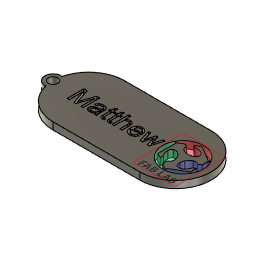
laser name tag v1 (Autodesk Fusion 360 design; units mm, degrees)
Autodesk Fusion 360 part; units mm, degrees
note: some values were not read from the file. Set by a fixed rule: which sketch regions a step uses.
sketch "Sketch1" plane through (0, 0, 0) normal (0, 0, 1) x (1, 0, 0)
  line L0 (15, -15) -> (51.5001, -15)
  arc A0 (51.5001, -15) -> (51.5001, 15) centre (51.5001, 0) ccw
  line L1 (51.5001, 15) -> (15, 15)
  line L2 (0, 0) -> (66.5001, 0) construction
  circle A1 centre (0, 0) radius 2
  line L3 (-3.4999, -0.0257) -> (-3.4999, 9)
  line L4 (15, -13.5) -> (51.5001, -13.5)
  arc A2 (51.5001, -13.5) -> (51.5001, 13.5) centre (51.5001, 0) ccw
  line L5 (51.5001, 13.5) -> (15, 13.5)
  arc A3 (0.4083, 3.4761) -> (0.4083, -3.4761) centre (0, 0) ccw
  arc A4 (15, 15) -> (0.4083, 3.4761) centre (15, 0) ccw
  arc A5 (0.4083, -3.4761) -> (15, -15) centre (15, 0) ccw
  arc A6 (15, 13.5) -> (1.5583, 1.2536) centre (15, 0) ccw
  arc A7 (1.5583, -1.2536) -> (15, -13.5) centre (15, 0) ccw
  dimension "d3" = 30
  dimension "d4" = 7
  dimension "d5" = 70
  constraint tangent L0 A0
  constraint tangent A0 L1
  constraint parallel L0 L1
  constraint tangent L1 A4
  constraint tangent L0 A4
  constraint midpoint A0 L2.end
  constraint horizontal L2
  constraint coincident L3.start A3
  constraint vertical L3
  constraint concentric A4 A5
  constraint coincident L2.start A4
  constraint concentric A0 A2
  constraint tangent L4 A6
  constraint tangent L4 A2
  constraint tangent A2 L5
  constraint tangent L5 A6
  constraint coincident A1 A6.end
  constraint concentric A6 A7
  constraint coincident A1 A7.start
  measures "d3" distance of L0 L1
  measures "d4" diameter of A3
  measures "d5" distance of L2.end L3
extrude "Extrude1" add sketch "Sketch1" along normal blind 3 contours L0 A0 L1 A3 A4 A5 | A1 L4 A2 L5 A6 A7
sketch "Sketch2" plane through (0, 0, 3) normal (0, 0, 1) x (-1, 0, 0)
  circle A0 centre (0, 0) radius 2
  arc A1 (3.4999, 0.0257) -> (-0.4083, 3.4761) centre (0, 0) ccw
  arc A2 (-0.4083, 3.4761) -> (-15, 15) centre (-15, 0) ccw
  line L0 (-15, 15) -> (-51.5001, 15)
  arc A3 (-51.5001, 15) -> (-51.5001, -15) centre (-51.5001, 0) ccw
  line L1 (-51.5001, -15) -> (-15, -15)
  arc A4 (-15, -15) -> (-0.4083, -3.4761) centre (-15, 0) ccw
  arc A5 (-0.4083, -3.4761) -> (3.4999, -0.0257) centre (0, 0) ccw
  line L2 (3.4999, -0.0257) -> (3.4999, 0.0257)
  line L3 (-1.75, 0) -> (-22.5, 0)
  line L4 (-9.4222, 3.5) -> (-9.4222, -3.5)
  line L5 (-9.4222, -3.5) -> (-10.8165, -3.5)
  line L6 (-10.8165, -3.5) -> (-12.4734, 1.4563)
  spline S0 degree 2 poles (-12.4734, 1.4563) (-12.7026, 2.1487) (-12.8076, 2.4925) knots 0 0 0 1 1 1
  spline S1 degree 2 poles (-12.8076, 2.4925) (-12.927, 2.1105) (-13.1801, 1.3704) knots 0 0 0 1 1 1
  line L7 (-13.1801, 1.3704) -> (-14.8561, -3.5)
  line L8 (-14.8561, -3.5) -> (-16.1023, -3.5)
  line L9 (-16.1023, -3.5) -> (-16.1023, 3.5)
  line L10 (-16.1023, 3.5) -> (-15.2094, 3.5)
  line L11 (-15.2094, 3.5) -> (-15.2094, -2.3588)
  line L12 (-15.2094, -2.3588) -> (-13.1753, 3.5)
  line L13 (-13.1753, 3.5) -> (-12.3397, 3.5)
  line L14 (-12.3397, 3.5) -> (-10.3151, -2.4591)
  line L15 (-10.3151, -2.4591) -> (-10.3151, 3.5)
  line L16 (-10.3151, 3.5) -> (-9.4222, 3.5)
  spline S2 degree 2 poles (-20.796, 2.8745) (-20.3186, 3.2804) (-19.8769, 3.4475) knots 0 0 0 1 1 1
  spline S3 degree 2 poles (-19.8769, 3.4475) (-19.4352, 3.6146) (-18.9291, 3.6146) knots 0 0 0 1 1 1
  spline S4 degree 2 poles (-18.9291, 3.6146) (-18.0935, 3.6146) (-17.6446, 3.2063) knots 0 0 0 1 1 1
  spline S5 degree 2 poles (-17.6446, 3.2063) (-17.1958, 2.7981) (-17.1958, 2.163) knots 0 0 0 1 1 1
  spline S6 degree 2 poles (-17.1958, 2.163) (-17.1958, 1.7906) (-17.3653, 1.4826) knots 0 0 0 1 1 1
  spline S7 degree 2 poles (-17.3653, 1.4826) (-17.5348, 1.1746) (-17.8093, 0.9884) knots 0 0 0 1 1 1
  spline S8 degree 2 poles (-17.8093, 0.9884) (-18.0839, 0.8022) (-18.4277, 0.7067) knots 0 0 0 1 1 1
  spline S9 degree 2 poles (-18.4277, 0.7067) (-18.6808, 0.6398) (-19.1917, 0.5778) knots 0 0 0 1 1 1
  spline S10 degree 2 poles (-19.1917, 0.5778) (-20.2326, 0.4536) (-20.7244, 0.2817) knots 0 0 0 1 1 1
  spline S11 degree 2 poles (-20.7244, 0.2817) (-20.7292, 0.105) (-20.7292, 0.0573) knots 0 0 0 1 1 1
  spline S12 degree 2 poles (-20.7292, 0.0573) (-20.7292, -0.4679) (-20.4857, -0.6828) knots 0 0 0 1 1 1
  spline S13 degree 2 poles (-20.4857, -0.6828) (-20.1562, -0.9741) (-19.5068, -0.9741) knots 0 0 0 1 1 1
  spline S14 degree 2 poles (-19.5068, -0.9741) (-18.9004, -0.9741) (-18.6115, -0.7616) knots 0 0 0 1 1 1
  spline S15 degree 2 poles (-18.6115, -0.7616) (-18.3226, -0.5491) (-18.1842, -0.0095) knots 0 0 0 1 1 1
  line L17 (-18.1842, -0.0095) -> (-17.3438, -0.1241)
  spline S16 degree 2 poles (-17.3438, -0.1241) (-17.4584, -0.6637) (-17.721, -0.9956) knots 0 0 0 1 1 1
  spline S17 degree 2 poles (-17.721, -0.9956) (-17.9836, -1.3274) (-18.4802, -1.5065) knots 0 0 0 1 1 1
  spline S18 degree 2 poles (-18.4802, -1.5065) (-18.9768, -1.6855) (-19.631, -1.6855) knots 0 0 0 1 1 1
  spline S19 degree 2 poles (-19.631, -1.6855) (-20.2804, -1.6855) (-20.6862, -1.5327) knots 0 0 0 1 1 1
  spline S20 degree 2 poles (-20.6862, -1.5327) (-21.0921, -1.3799) (-21.2831, -1.1484) knots 0 0 0 1 1 1
  spline S21 degree 2 poles (-21.2831, -1.1484) (-21.4741, -0.9168) (-21.5505, -0.5634) knots 0 0 0 1 1 1
  spline S22 degree 2 poles (-21.5505, -0.5634) (-21.5935, -0.3438) (-21.5935, 0.2292) knots 0 0 0 1 1 1
  line L18 (-21.5935, 0.2292) -> (-21.5935, 1.1)
  spline S23 degree 2 poles (-21.6484, 2.8912) (-21.7033, 3.2087) (-21.8656, 3.5) knots 0 0 0 1 1 1
  line L19 (-21.8656, 3.5) -> (-20.9679, 3.5)
  spline S24 degree 2 poles (-20.9679, 3.5) (-20.8342, 3.2326) (-20.796, 2.8745) knots 0 0 0 1 1 1
  spline S25 degree 2 poles (-20.7244, 0.955) (-20.2565, 1.146) (-19.3206, 1.2797) knots 0 0 0 1 1 1
  spline S26 degree 2 poles (-19.3206, 1.2797) (-18.7906, 1.3561) (-18.5709, 1.4516) knots 0 0 0 1 1 1
  spline S27 degree 2 poles (-18.5709, 1.4516) (-18.3513, 1.5471) (-18.2319, 1.7309) knots 0 0 0 1 1 1
  spline S28 degree 2 poles (-18.2319, 1.7309) (-18.1126, 1.9147) (-18.1126, 2.1392) knots 0 0 0 1 1 1
  spline S29 degree 2 poles (-18.1126, 2.1392) (-18.1126, 2.4829) (-18.3728, 2.7121) knots 0 0 0 1 1 1
  spline S30 degree 2 poles (-18.3728, 2.7121) (-18.633, 2.9413) (-19.1344, 2.9413) knots 0 0 0 1 1 1
  spline S31 degree 2 poles (-19.1344, 2.9413) (-19.631, 2.9413) (-20.0177, 2.7241) knots 0 0 0 1 1 1
  spline S32 degree 2 poles (-20.0177, 2.7241) (-20.4045, 2.5068) (-20.5859, 2.1296) knots 0 0 0 1 1 1
  line L20 (-20.7244, 1.1) -> (-20.7244, 0.955)
  line L21 (-24.8022, 2.7312) -> (-24.9263, 3.4905)
  spline S33 degree 2 poles (-24.9263, 3.4905) (-24.5634, 3.5668) (-24.2769, 3.5668) knots 0 0 0 1 1 1
  spline S34 degree 2 poles (-24.2769, 3.5668) (-23.809, 3.5668) (-23.5512, 3.4188) knots 0 0 0 1 1 1
  spline S35 degree 2 poles (-23.5512, 3.4188) (-23.2933, 3.2708) (-23.1883, 3.0297) knots 0 0 0 1 1 1
  spline S36 degree 2 poles (-23.1883, 3.0297) (-23.0832, 2.7885) (-23.0832, 2.015) knots 0 0 0 1 1 1
  line L22 (-23.0832, 2.015) -> (-23.0832, -0.9025)
  line L23 (-23.0832, -0.9025) -> (-22.4529, -0.9025)
  line L24 (-22.4529, -0.9025) -> (-22.4529, -1.5709)
  line L25 (-22.4529, -1.5709) -> (-23.0832, -1.5709)
  line L26 (-23.0832, -1.5709) -> (-23.0832, -2.8267)
  line L27 (-23.0832, -2.8267) -> (-23.9379, -3.3424)
  line L28 (-23.9379, -3.3424) -> (-23.9379, -1.5709)
  line L29 (-23.9379, -1.5709) -> (-24.8022, -1.5709)
  line L30 (-24.8022, -1.5709) -> (-24.8022, -0.9025)
  line L31 (-24.8022, -0.9025) -> (-23.9379, -0.9025)
  line L32 (-23.9379, -0.9025) -> (-23.9379, 2.0628)
  spline S37 degree 2 poles (-23.9379, 2.0628) (-23.9379, 2.4304) (-23.9833, 2.5355) knots 0 0 0 1 1 1
  spline S38 degree 2 poles (-23.9833, 2.5355) (-24.0286, 2.6405) (-24.1313, 2.7026) knots 0 0 0 1 1 1
  spline S39 degree 2 poles (-24.1313, 2.7026) (-24.234, 2.7647) (-24.425, 2.7647) knots 0 0 0 1 1 1
  spline S40 degree 2 poles (-24.425, 2.7647) (-24.5682, 2.7647) (-24.8022, 2.7312) knots 0 0 0 1 1 1
  line L33 (-27.5191, 2.7312) -> (-27.6432, 3.4905)
  spline S41 degree 2 poles (-27.6432, 3.4905) (-27.2804, 3.5668) (-26.9939, 3.5668) knots 0 0 0 1 1 1
  spline S42 degree 2 poles (-26.9939, 3.5668) (-26.5259, 3.5668) (-26.2681, 3.4188) knots 0 0 0 1 1 1
  spline S43 degree 2 poles (-26.2681, 3.4188) (-26.0102, 3.2708) (-25.9052, 3.0297) knots 0 0 0 1 1 1
  spline S44 degree 2 poles (-25.9052, 3.0297) (-25.8001, 2.7885) (-25.8001, 2.015) knots 0 0 0 1 1 1
  line L34 (-25.8001, 2.015) -> (-25.8001, -0.9025)
  line L35 (-25.8001, -0.9025) -> (-25.1698, -0.9025)
  line L36 (-25.1698, -0.9025) -> (-25.1698, -1.5709)
  line L37 (-25.1698, -1.5709) -> (-25.8001, -1.5709)
  line L38 (-25.8001, -1.5709) -> (-25.8001, -2.8267)
  line L39 (-25.8001, -2.8267) -> (-26.6548, -3.3424)
  line L40 (-26.6548, -3.3424) -> (-26.6548, -1.5709)
  line L41 (-26.6548, -1.5709) -> (-27.5191, -1.5709)
  line L42 (-27.5191, -1.5709) -> (-27.5191, -0.9025)
  line L43 (-27.5191, -0.9025) -> (-26.6548, -0.9025)
  line L44 (-26.6548, -0.9025) -> (-26.6548, 2.0628)
  spline S45 degree 2 poles (-26.6548, 2.0628) (-26.6548, 2.4304) (-26.7002, 2.5355) knots 0 0 0 1 1 1
  spline S46 degree 2 poles (-26.7002, 2.5355) (-26.7456, 2.6405) (-26.8482, 2.7026) knots 0 0 0 1 1 1
  spline S47 degree 2 poles (-26.8482, 2.7026) (-26.9509, 2.7647) (-27.1419, 2.7647) knots 0 0 0 1 1 1
  spline S48 degree 2 poles (-27.1419, 2.7647) (-27.2851, 2.7647) (-27.5191, 2.7312) knots 0 0 0 1 1 1
  line L45 (-28.3595, 3.5) -> (-28.3595, -3.5)
  line L46 (-28.3595, -3.5) -> (-29.219, -3.5)
  line L47 (-29.219, -3.5) -> (-29.219, -0.9884)
  spline S49 degree 2 poles (-29.219, -0.9884) (-29.8206, -1.6855) (-30.7374, -1.6855) knots 0 0 0 1 1 1
  spline S50 degree 2 poles (-30.7374, -1.6855) (-31.3008, -1.6855) (-31.7162, -1.4635) knots 0 0 0 1 1 1
  spline S51 degree 2 poles (-31.7162, -1.4635) (-32.1317, -1.2415) (-32.3107, -0.8499) knots 0 0 0 1 1 1
  spline S52 degree 2 poles (-32.3107, -0.8499) (-32.4898, -0.4584) (-32.4898, 0.2865) knots 0 0 0 1 1 1
  line L48 (-32.4898, 0.2865) -> (-32.4898, 3.5)
  line L49 (-32.4898, 3.5) -> (-31.6303, 3.5)
  line L50 (-31.6303, 3.5) -> (-31.6303, 0.2865)
  spline S53 degree 2 poles (-31.6303, 0.2865) (-31.6303, -0.3581) (-31.351, -0.6518) knots 0 0 0 1 1 1
  spline S54 degree 2 poles (-31.351, -0.6518) (-31.0716, -0.9454) (-30.5607, -0.9454) knots 0 0 0 1 1 1
  spline S55 degree 2 poles (-30.5607, -0.9454) (-30.1787, -0.9454) (-29.8421, -0.7473) knots 0 0 0 1 1 1
  spline S56 degree 2 poles (-29.8421, -0.7473) (-29.5055, -0.5491) (-29.3622, -0.2101) knots 0 0 0 1 1 1
  spline S57 degree 2 poles (-29.3622, -0.2101) (-29.219, 0.1289) (-29.219, 0.7258) knots 0 0 0 1 1 1
  line L51 (-29.219, 0.7258) -> (-29.219, 3.5)
  line L52 (-29.219, 3.5) -> (-28.3595, 3.5)
  line L53 (-37.2694, 1.867) -> (-38.1576, 1.9768)
  spline S58 degree 2 poles (-38.1576, 1.9768) (-37.9475, 2.7551) (-37.3793, 3.1849) knots 0 0 0 1 1 1
  spline S59 degree 2 poles (-37.3793, 3.1849) (-36.8111, 3.6146) (-35.9277, 3.6146) knots 0 0 0 1 1 1
  spline S60 degree 2 poles (-35.9277, 3.6146) (-34.8151, 3.6146) (-34.1634, 2.9294) knots 0 0 0 1 1 1
  spline S61 degree 2 poles (-34.1634, 2.9294) (-33.5116, 2.2442) (-33.5116, 1.0075) knots 0 0 0 1 1 1
  spline S62 degree 2 poles (-33.5116, 1.0075) (-33.5116, -0.2722) (-34.1705, -0.9789) knots 0 0 0 1 1 1
  spline S63 degree 2 poles (-34.1705, -0.9789) (-34.8295, -1.6855) (-35.8799, -1.6855) knots 0 0 0 1 1 1
  spline S64 degree 2 poles (-35.8799, -1.6855) (-36.897, -1.6855) (-37.5416, -0.9932) knots 0 0 0 1 1 1
  spline S65 degree 2 poles (-37.5416, -0.9932) (-38.1862, -0.3008) (-38.1862, 0.955) knots 0 0 0 1 1 1
  spline S66 degree 2 poles (-38.1862, 0.955) (-38.1862, 1.0314) (-38.1814, 1.1842) knots 0 0 0 1 1 1
  spline S67 degree 2 poles (-34.3997, 1.1842) (-34.4475, 2.0198) (-34.8724, 2.4638) knots 0 0 0 1 1 1
  spline S68 degree 2 poles (-34.8724, 2.4638) (-35.2974, 2.9079) (-35.9325, 2.9079) knots 0 0 0 1 1 1
  spline S69 degree 2 poles (-35.9325, 2.9079) (-36.4052, 2.9079) (-36.7394, 2.6596) knots 0 0 0 1 1 1
  spline S70 degree 2 poles (-36.7394, 2.6596) (-37.0737, 2.4113) (-37.2694, 1.867) knots 0 0 0 1 1 1
  spline S71 degree 2 poles (-37.279, 0.4775) (-37.2217, -0.1623) (-36.9543, -0.4823) knots 0 0 0 1 1 1
  spline S72 degree 2 poles (-36.9543, -0.4823) (-36.5437, -0.9789) (-35.8895, -0.9789) knots 0 0 0 1 1 1
  spline S73 degree 2 poles (-35.8895, -0.9789) (-35.2974, -0.9789) (-34.8939, -0.5825) knots 0 0 0 1 1 1
  spline S74 degree 2 poles (-34.8939, -0.5825) (-34.4905, -0.1862) (-34.4475, 0.4775) knots 0 0 0 1 1 1
  line L54 (-40.1726, 3.5) -> (-38.6207, -1.5709)
  line L55 (-38.6207, -1.5709) -> (-39.5089, -1.5709)
  line L56 (-39.5089, -1.5709) -> (-40.3158, 1.3561)
  line L57 (-40.3158, 1.3561) -> (-40.6166, 2.4447)
  spline S75 degree 2 poles (-40.6166, 2.4447) (-40.6357, 2.3636) (-40.8793, 1.399) knots 0 0 0 1 1 1
  line L58 (-40.8793, 1.399) -> (-41.6862, -1.5709)
  line L59 (-41.6862, -1.5709) -> (-42.5696, -1.5709)
  line L60 (-42.5696, -1.5709) -> (-43.3288, 1.3704)
  line L61 (-43.3288, 1.3704) -> (-43.5819, 2.3397)
  line L62 (-43.5819, 2.3397) -> (-43.8731, 1.3608)
  line L63 (-43.8731, 1.3608) -> (-44.7422, -1.5709)
  line L64 (-44.7422, -1.5709) -> (-45.5778, -1.5709)
  line L65 (-45.5778, -1.5709) -> (-43.9925, 3.5)
  line L66 (-43.9925, 3.5) -> (-43.0996, 3.5)
  line L67 (-43.0996, 3.5) -> (-42.2926, 0.4632)
  line L68 (-42.2926, 0.4632) -> (-42.0969, -0.4011)
  line L69 (-42.0969, -0.4011) -> (-41.0703, 3.5)
  line L70 (-41.0703, 3.5) -> (-40.1726, 3.5)
  line L71 (-20.7244, 1.1) -> (-21.5935, 1.1)
  line L72 (-21.5935, 1.4) -> (-20.7225, 1.4)
  spline S76 degree 2 poles (-20.5859, 2.1296) (-20.7081, 1.8726) (-20.7225, 1.4) knots 0 0 0 0.88234 0.88234 0.88234
  spline S77 degree 2 poles (-21.5935, 1.4) (-21.594, 2.577) (-21.6484, 2.8912) knots 0.010398 0.010398 0.010398 1 1 1
  line L73 (-35.9, 0.4775) -> (-35.9, 1.1842)
  line L74 (-35.7, 1.1842) -> (-35.7, 0.4775)
  line L75 (-34.4475, 0.4775) -> (-35.7, 0.4775)
  line L76 (-35.9, 0.4775) -> (-37.279, 0.4775)
  line L77 (-38.1814, 1.1842) -> (-35.9, 1.1842)
  line L78 (-35.7, 1.1842) -> (-34.3997, 1.1842)
  constraint horizontal L71
  constraint horizontal L72
  constraint vertical L73
  constraint vertical L74
  constraint collinear L75 L76
  constraint coincident L74.start L77
  constraint collinear L77 L78
extrude "Extrude2" cut sketch "Sketch2" against normal blind 3 contours L3 L4 L5 L6 L14 L15 | L3 L4 L15 L16 | L3 L6 S0 S1 L7 L12 L13 L14 | L3 L7 L8 L9 L11 L12 | L3 L9 L10 L11 | L3 S12 S13 S14 S15 L17 S16 S17 S18 S19 S20 S21 S22 | L3 S2 S3 S4 S5 S6 S7 S8 S9 S10 S11 S12 S22 L18 S23 L19 S24 S25 S26 S27 S28 S29 S30 S31 S32 L20 L71 L72 S76 S77 | L21 S33 S34 S35 S36 L22 L23 L24 L25 L26 L27 L28 L29 L30 L31 L32 S37 S38 S39 S40 | L33 S41 S42 S43 S44 L34 L35 L36 L37 L38 L39 L40 L41 L42 L43 L44 S45 S46 S47 S48 | L45 L46 L47 S49 S50 S51 S52 L48 L49 L50 S53 S54 S55 S56 S57 L51 L52 | L53 S58 S59 S60 S61 S62 S63 S64 S65 S66 S67 S68 S69 S70 S71 S72 S73 S74 L73 L74 L75 L76 L77 L78 | L54 L55 L56 L57 S75 L58 L59 L60 L61 L62 L63 L64 L65 L66 L67 L68 L69 L70
sketch "Sketch3" plane through (0, 0, 3) normal (0, 0, 1) x (-1, 0, 0)
  spline S0 degree 2 poles (-29.3622, -0.2101) (-29.219, 0.1289) (-29.219, 0.7258) knots 0 0 0 1 1 1
  line L0 (-29.219, 0.7258) -> (-29.219, 3.5)
  line L1 (-29.219, 3.5) -> (-28.3595, 3.5)
  line L2 (-28.3595, 3.5) -> (-28.3595, -3.5)
  line L3 (-28.3595, -3.5) -> (-29.219, -3.5)
  line L4 (-29.219, -3.5) -> (-29.219, -0.9884)
  spline S1 degree 2 poles (-29.219, -0.9884) (-29.8206, -1.6855) (-30.7374, -1.6855) knots 0 0 0 1 1 1
  spline S2 degree 2 poles (-30.7374, -1.6855) (-31.3008, -1.6855) (-31.7162, -1.4635) knots 0 0 0 1 1 1
  spline S3 degree 2 poles (-31.7162, -1.4635) (-32.1317, -1.2415) (-32.3107, -0.8499) knots 0 0 0 1 1 1
  spline S4 degree 2 poles (-32.3107, -0.8499) (-32.4898, -0.4584) (-32.4898, 0.2865) knots 0 0 0 1 1 1
  line L5 (-32.4898, 0.2865) -> (-32.4898, 3.5)
  line L6 (-32.4898, 3.5) -> (-31.6303, 3.5)
  line L7 (-31.6303, 3.5) -> (-31.6303, 0.2865)
  spline S5 degree 2 poles (-31.6303, 0.2865) (-31.6303, -0.3581) (-31.351, -0.6518) knots 0 0 0 1 1 1
  spline S6 degree 2 poles (-31.351, -0.6518) (-31.0716, -0.9454) (-30.5607, -0.9454) knots 0 0 0 1 1 1
  spline S7 degree 2 poles (-30.5607, -0.9454) (-30.1787, -0.9454) (-29.8421, -0.7473) knots 0 0 0 1 1 1
  spline S8 degree 2 poles (-29.8421, -0.7473) (-29.5055, -0.5491) (-29.3622, -0.2101) knots 0 0 0 1 1 1
  line L8 (-12.3397, 3.5) -> (-10.3151, -2.4591)
  line L9 (-10.3151, -2.4591) -> (-10.3151, 3.5)
  line L10 (-10.3151, 3.5) -> (-9.4222, 3.5)
  line L11 (-9.4222, 3.5) -> (-9.4222, -3.5)
  line L12 (-9.4222, -3.5) -> (-10.8165, -3.5)
  line L13 (-10.8165, -3.5) -> (-12.4734, 1.4563)
  spline S9 degree 2 poles (-12.4734, 1.4563) (-12.7026, 2.1487) (-12.8076, 2.4925) knots 0 0 0 1 1 1
  spline S10 degree 2 poles (-12.8076, 2.4925) (-12.927, 2.1105) (-13.1801, 1.3704) knots 0 0 0 1 1 1
  line L14 (-13.1801, 1.3704) -> (-14.8561, -3.5)
  line L15 (-14.8561, -3.5) -> (-16.1023, -3.5)
  line L16 (-16.1023, -3.5) -> (-16.1023, 3.5)
  line L17 (-16.1023, 3.5) -> (-15.2094, 3.5)
  line L18 (-15.2094, 3.5) -> (-15.2094, -2.3588)
  line L19 (-15.2094, -2.3588) -> (-13.1753, 3.5)
  line L20 (-13.1753, 3.5) -> (-12.3397, 3.5)
  spline S11 degree 2 poles (-26.7002, 2.5355) (-26.7456, 2.6405) (-26.8482, 2.7026) knots 0 0 0 1 1 1
  spline S12 degree 2 poles (-26.8482, 2.7026) (-26.9509, 2.7647) (-27.1419, 2.7647) knots 0 0 0 1 1 1
  spline S13 degree 2 poles (-27.1419, 2.7647) (-27.2851, 2.7647) (-27.5191, 2.7312) knots 0 0 0 1 1 1
  line L21 (-27.5191, 2.7312) -> (-27.6432, 3.4905)
  spline S14 degree 2 poles (-27.6432, 3.4905) (-27.2804, 3.5668) (-26.9939, 3.5668) knots 0 0 0 1 1 1
  spline S15 degree 2 poles (-26.9939, 3.5668) (-26.5259, 3.5668) (-26.2681, 3.4188) knots 0 0 0 1 1 1
  spline S16 degree 2 poles (-26.2681, 3.4188) (-26.0102, 3.2708) (-25.9052, 3.0297) knots 0 0 0 1 1 1
  spline S17 degree 2 poles (-25.9052, 3.0297) (-25.8001, 2.7885) (-25.8001, 2.015) knots 0 0 0 1 1 1
  line L22 (-25.8001, 2.015) -> (-25.8001, -0.9025)
  line L23 (-25.8001, -0.9025) -> (-25.1698, -0.9025)
  line L24 (-25.1698, -0.9025) -> (-25.1698, -1.5709)
  line L25 (-25.1698, -1.5709) -> (-25.8001, -1.5709)
  line L26 (-25.8001, -1.5709) -> (-25.8001, -2.8267)
  line L27 (-25.8001, -2.8267) -> (-26.6548, -3.3424)
  line L28 (-26.6548, -3.3424) -> (-26.6548, -1.5709)
  line L29 (-26.6548, -1.5709) -> (-27.5191, -1.5709)
  line L30 (-27.5191, -1.5709) -> (-27.5191, -0.9025)
  line L31 (-27.5191, -0.9025) -> (-26.6548, -0.9025)
  line L32 (-26.6548, -0.9025) -> (-26.6548, 2.0628)
  spline S18 degree 2 poles (-26.6548, 2.0628) (-26.6548, 2.4304) (-26.7002, 2.5355) knots 0 0 0 1 1 1
  line L33 (-38.1814, 1.1842) -> (-35.9, 1.1842)
  line L34 (-35.9, 1.1842) -> (-35.9, 0.4775)
  line L35 (-35.9, 0.4775) -> (-37.279, 0.4775)
  spline S19 degree 2 poles (-37.279, 0.4775) (-37.2217, -0.1623) (-36.9543, -0.4823) knots 0 0 0 1 1 1
  spline S20 degree 2 poles (-36.9543, -0.4823) (-36.5437, -0.9789) (-35.8895, -0.9789) knots 0 0 0 1 1 1
  spline S21 degree 2 poles (-35.8895, -0.9789) (-35.2974, -0.9789) (-34.8939, -0.5825) knots 0 0 0 1 1 1
  spline S22 degree 2 poles (-34.8939, -0.5825) (-34.4905, -0.1862) (-34.4475, 0.4775) knots 0 0 0 1 1 1
  line L36 (-34.4475, 0.4775) -> (-35.7, 0.4775)
  line L37 (-35.7, 0.4775) -> (-35.7, 1.1842)
  line L38 (-35.7, 1.1842) -> (-34.3997, 1.1842)
  spline S23 degree 2 poles (-34.3997, 1.1842) (-34.4475, 2.0198) (-34.8724, 2.4638) knots 0 0 0 1 1 1
  spline S24 degree 2 poles (-34.8724, 2.4638) (-35.2974, 2.9079) (-35.9325, 2.9079) knots 0 0 0 1 1 1
  spline S25 degree 2 poles (-35.9325, 2.9079) (-36.4052, 2.9079) (-36.7394, 2.6596) knots 0 0 0 1 1 1
  spline S26 degree 2 poles (-36.7394, 2.6596) (-37.0737, 2.4113) (-37.2694, 1.867) knots 0 0 0 1 1 1
  line L39 (-37.2694, 1.867) -> (-38.1576, 1.9768)
  spline S27 degree 2 poles (-38.1576, 1.9768) (-37.9475, 2.7551) (-37.3793, 3.1849) knots 0 0 0 1 1 1
  spline S28 degree 2 poles (-37.3793, 3.1849) (-36.8111, 3.6146) (-35.9277, 3.6146) knots 0 0 0 1 1 1
  spline S29 degree 2 poles (-35.9277, 3.6146) (-34.8151, 3.6146) (-34.1634, 2.9294) knots 0 0 0 1 1 1
  spline S30 degree 2 poles (-34.1634, 2.9294) (-33.5116, 2.2442) (-33.5116, 1.0075) knots 0 0 0 1 1 1
  spline S31 degree 2 poles (-33.5116, 1.0075) (-33.5116, -0.2722) (-34.1705, -0.9789) knots 0 0 0 1 1 1
  spline S32 degree 2 poles (-34.1705, -0.9789) (-34.8295, -1.6855) (-35.8799, -1.6855) knots 0 0 0 1 1 1
  spline S33 degree 2 poles (-35.8799, -1.6855) (-36.897, -1.6855) (-37.5416, -0.9932) knots 0 0 0 1 1 1
  spline S34 degree 2 poles (-37.5416, -0.9932) (-38.1862, -0.3008) (-38.1862, 0.955) knots 0 0 0 1 1 1
  spline S35 degree 2 poles (-38.1862, 0.955) (-38.1862, 1.0314) (-38.1814, 1.1842) knots 0 0 0 1 1 1
  line L40 (-21.5935, 0.2292) -> (-21.5935, 1.1)
  line L41 (-21.5935, 1.1) -> (-20.7244, 1.1)
  line L42 (-20.7244, 1.1) -> (-20.7244, 0.955)
  spline S36 degree 2 poles (-20.7244, 0.955) (-20.2565, 1.146) (-19.3206, 1.2797) knots 0 0 0 1 1 1
  spline S37 degree 2 poles (-19.3206, 1.2797) (-18.7906, 1.3561) (-18.5709, 1.4516) knots 0 0 0 1 1 1
  spline S38 degree 2 poles (-18.5709, 1.4516) (-18.3513, 1.5471) (-18.2319, 1.7309) knots 0 0 0 1 1 1
  spline S39 degree 2 poles (-18.2319, 1.7309) (-18.1126, 1.9147) (-18.1126, 2.1392) knots 0 0 0 1 1 1
  spline S40 degree 2 poles (-18.1126, 2.1392) (-18.1126, 2.4829) (-18.3728, 2.7121) knots 0 0 0 1 1 1
  spline S41 degree 2 poles (-18.3728, 2.7121) (-18.633, 2.9413) (-19.1344, 2.9413) knots 0 0 0 1 1 1
  spline S42 degree 2 poles (-19.1344, 2.9413) (-19.631, 2.9413) (-20.0177, 2.7241) knots 0 0 0 1 1 1
  spline S43 degree 2 poles (-20.0177, 2.7241) (-20.4045, 2.5068) (-20.5859, 2.1296) knots 0 0 0 1 1 1
  spline S44 degree 2 poles (-20.5859, 2.1296) (-20.7081, 1.8726) (-20.7225, 1.4) knots 0 0 0 0.88234 0.88234 0.88234
  line L43 (-20.7225, 1.4) -> (-21.5935, 1.4)
  spline S45 degree 2 poles (-21.5935, 1.4) (-21.594, 2.577) (-21.6484, 2.8912) knots 0.010398 0.010398 0.010398 1 1 1
  spline S46 degree 2 poles (-21.6484, 2.8912) (-21.7033, 3.2087) (-21.8656, 3.5) knots 0 0 0 1 1 1
  line L44 (-21.8656, 3.5) -> (-20.9679, 3.5)
  spline S47 degree 2 poles (-20.9679, 3.5) (-20.8342, 3.2326) (-20.796, 2.8745) knots 0 0 0 1 1 1
  spline S48 degree 2 poles (-20.796, 2.8745) (-20.3186, 3.2804) (-19.8769, 3.4475) knots 0 0 0 1 1 1
  spline S49 degree 2 poles (-19.8769, 3.4475) (-19.4352, 3.6146) (-18.9291, 3.6146) knots 0 0 0 1 1 1
  spline S50 degree 2 poles (-18.9291, 3.6146) (-18.0935, 3.6146) (-17.6446, 3.2063) knots 0 0 0 1 1 1
  spline S51 degree 2 poles (-17.6446, 3.2063) (-17.1958, 2.7981) (-17.1958, 2.163) knots 0 0 0 1 1 1
  spline S52 degree 2 poles (-17.1958, 2.163) (-17.1958, 1.7906) (-17.3653, 1.4826) knots 0 0 0 1 1 1
  spline S53 degree 2 poles (-17.3653, 1.4826) (-17.5348, 1.1746) (-17.8093, 0.9884) knots 0 0 0 1 1 1
  spline S54 degree 2 poles (-17.8093, 0.9884) (-18.0839, 0.8022) (-18.4277, 0.7067) knots 0 0 0 1 1 1
  spline S55 degree 2 poles (-18.4277, 0.7067) (-18.6808, 0.6398) (-19.1917, 0.5778) knots 0 0 0 1 1 1
  spline S56 degree 2 poles (-19.1917, 0.5778) (-20.2326, 0.4536) (-20.7244, 0.2817) knots 0 0 0 1 1 1
  spline S57 degree 2 poles (-20.7244, 0.2817) (-20.7292, 0.105) (-20.7292, 0.0573) knots 0 0 0 1 1 1
  spline S58 degree 2 poles (-20.7292, 0.0573) (-20.7292, -0.4679) (-20.4857, -0.6828) knots 0 0 0 1 1 1
  spline S59 degree 2 poles (-20.4857, -0.6828) (-20.1562, -0.9741) (-19.5068, -0.9741) knots 0 0 0 1 1 1
  spline S60 degree 2 poles (-19.5068, -0.9741) (-18.9004, -0.9741) (-18.6115, -0.7616) knots 0 0 0 1 1 1
  spline S61 degree 2 poles (-18.6115, -0.7616) (-18.3226, -0.5491) (-18.1842, -0.0095) knots 0 0 0 1 1 1
  line L45 (-18.1842, -0.0095) -> (-17.3438, -0.1241)
  spline S62 degree 2 poles (-17.3438, -0.1241) (-17.4584, -0.6637) (-17.721, -0.9956) knots 0 0 0 1 1 1
  spline S63 degree 2 poles (-17.721, -0.9956) (-17.9836, -1.3274) (-18.4802, -1.5065) knots 0 0 0 1 1 1
  spline S64 degree 2 poles (-18.4802, -1.5065) (-18.9768, -1.6855) (-19.631, -1.6855) knots 0 0 0 1 1 1
  spline S65 degree 2 poles (-19.631, -1.6855) (-20.2804, -1.6855) (-20.6862, -1.5327) knots 0 0 0 1 1 1
  spline S66 degree 2 poles (-20.6862, -1.5327) (-21.0921, -1.3799) (-21.2831, -1.1484) knots 0 0 0 1 1 1
  spline S67 degree 2 poles (-21.2831, -1.1484) (-21.4741, -0.9168) (-21.5505, -0.5634) knots 0 0 0 1 1 1
  spline S68 degree 2 poles (-21.5505, -0.5634) (-21.5935, -0.3438) (-21.5935, 0.2292) knots 0 0 0 1 1 1
  spline S69 degree 2 poles (-23.9833, 2.5355) (-24.0286, 2.6405) (-24.1313, 2.7026) knots 0 0 0 1 1 1
  spline S70 degree 2 poles (-24.1313, 2.7026) (-24.234, 2.7647) (-24.425, 2.7647) knots 0 0 0 1 1 1
  spline S71 degree 2 poles (-24.425, 2.7647) (-24.5682, 2.7647) (-24.8022, 2.7312) knots 0 0 0 1 1 1
  line L46 (-24.8022, 2.7312) -> (-24.9263, 3.4905)
  spline S72 degree 2 poles (-24.9263, 3.4905) (-24.5634, 3.5668) (-24.2769, 3.5668) knots 0 0 0 1 1 1
  spline S73 degree 2 poles (-24.2769, 3.5668) (-23.809, 3.5668) (-23.5512, 3.4188) knots 0 0 0 1 1 1
  spline S74 degree 2 poles (-23.5512, 3.4188) (-23.2933, 3.2708) (-23.1883, 3.0297) knots 0 0 0 1 1 1
  spline S75 degree 2 poles (-23.1883, 3.0297) (-23.0832, 2.7885) (-23.0832, 2.015) knots 0 0 0 1 1 1
  line L47 (-23.0832, 2.015) -> (-23.0832, -0.9025)
  line L48 (-23.0832, -0.9025) -> (-22.4529, -0.9025)
  line L49 (-22.4529, -0.9025) -> (-22.4529, -1.5709)
  line L50 (-22.4529, -1.5709) -> (-23.0832, -1.5709)
  line L51 (-23.0832, -1.5709) -> (-23.0832, -2.8267)
  line L52 (-23.0832, -2.8267) -> (-23.9379, -3.3424)
  line L53 (-23.9379, -3.3424) -> (-23.9379, -1.5709)
  line L54 (-23.9379, -1.5709) -> (-24.8022, -1.5709)
  line L55 (-24.8022, -1.5709) -> (-24.8022, -0.9025)
  line L56 (-24.8022, -0.9025) -> (-23.9379, -0.9025)
  line L57 (-23.9379, -0.9025) -> (-23.9379, 2.0628)
  spline S76 degree 2 poles (-23.9379, 2.0628) (-23.9379, 2.4304) (-23.9833, 2.5355) knots 0 0 0 1 1 1
  line L58 (-42.2926, 0.4632) -> (-42.0969, -0.4011)
  line L59 (-42.0969, -0.4011) -> (-41.0703, 3.5)
  line L60 (-41.0703, 3.5) -> (-40.1726, 3.5)
  line L61 (-40.1726, 3.5) -> (-38.6207, -1.5709)
  line L62 (-38.6207, -1.5709) -> (-39.5089, -1.5709)
  line L63 (-39.5089, -1.5709) -> (-40.3158, 1.3561)
  line L64 (-40.3158, 1.3561) -> (-40.6166, 2.4447)
  spline S77 degree 2 poles (-40.6166, 2.4447) (-40.6357, 2.3636) (-40.8793, 1.399) knots 0 0 0 1 1 1
  line L65 (-40.8793, 1.399) -> (-41.6862, -1.5709)
  line L66 (-41.6862, -1.5709) -> (-42.5696, -1.5709)
  line L67 (-42.5696, -1.5709) -> (-43.3288, 1.3704)
  line L68 (-43.3288, 1.3704) -> (-43.5819, 2.3397)
  line L69 (-43.5819, 2.3397) -> (-43.8731, 1.3608)
  line L70 (-43.8731, 1.3608) -> (-44.7422, -1.5709)
  line L71 (-44.7422, -1.5709) -> (-45.5778, -1.5709)
  line L72 (-45.5778, -1.5709) -> (-43.9925, 3.5)
  line L73 (-43.9925, 3.5) -> (-43.0996, 3.5)
  line L74 (-43.0996, 3.5) -> (-42.2926, 0.4632)
  circle A0 centre (0, 0) radius 2
  arc A1 (3.4999, 0.0257) -> (-0.4083, 3.4761) centre (0, 0) ccw
  arc A2 (-0.4083, 3.4761) -> (-15, 15) centre (-15, 0) ccw
  line L75 (-15, 15) -> (-51.5001, 15)
  arc A3 (-51.5001, 15) -> (-51.5001, -15) centre (-51.5001, 0) ccw
  line L76 (-51.5001, -15) -> (-15, -15)
  arc A4 (-15, -15) -> (-0.4083, -3.4761) centre (-15, 0) ccw
  arc A5 (-0.4083, -3.4761) -> (3.4999, -0.0257) centre (0, 0) ccw
  line L77 (3.4999, -0.0257) -> (3.4999, 0.0257)
  circle A6 centre (-55.2374, 0.5704) radius 8.5704
  line L78 (-48.8, -3.5) -> (-48.008, -4.0325)
  line L79 (-48.8, -3.5) -> (-50.8419, -4.7509)
  line L80 (-50.8419, -4.7509) -> (-52.1863, -3.9664)
  line L81 (-54.1328, -5.3812) -> (-53.1818, -6.0261)
  line L82 (-53.1818, -6.0261) -> (-55.3282, -7.3191)
  line L83 (-55.3282, -7.3191) -> (-61.819, -3.4918)
  line L84 (-61.819, -3.4918) -> (-62.5353, -3.9233)
  ellipse E0 centre (-55.135, -3.5103) end of major axis (-58.1649, -3.5103) minor radius 1.9824 (-52.1863, -3.9664) -> (-54.1328, -5.3812) ccw
  line L85 (-62.774, -3.5103) -> (-62.0605, -3.0399)
  line L86 (-62.0605, -3.0399) -> (-62.0605, -0.6586)
  line L87 (-62.0605, -0.6586) -> (-60.7945, 0.1762)
  line L88 (-55.6013, 9.133) -> (-55.5731, 9.133)
  line L89 (-55.5731, 9.133) -> (-55.5731, 8.3003)
  line L90 (-55.5731, 8.3003) -> (-55.6013, 8.3003)
  line L91 (-55.6013, 8.3003) -> (-55.6013, 9.133)
  line L92 (-55.6013, 8.3003) -> (-62.1327, 4.4372)
  line L93 (-62.1327, 4.4372) -> (-62.1327, 1.7667)
  line L94 (-62.1327, 1.7667) -> (-60.9329, 2.4763)
  arc A7 (-60.7945, 0.1762) -> (-58.6848, -0.2431) centre (-59.4589, 1.379) ccw
  arc A8 (-58.6848, -0.2431) -> (-56.9518, 1.5465) centre (-60.9005, 3.6364) ccw
  arc A9 (-56.9518, 1.5465) -> (-56.5, 3.2) centre (-60.7439, 3.4711) ccw
  arc A10 (-56.5, 3.2) -> (-57.2, 5) centre (-58.3875, 3.5021) ccw
  arc A11 (-57.2, 5) -> (-59.0174, 5.0449) centre (-58.15, 3.35) ccw
  arc A12 (-59.0174, 5.0449) -> (-59.2259, 4.941) centre (-55.5904, -2.0964) ccw
  arc A13 (-59.2259, 4.941) -> (-60.9329, 2.4763) centre (-57.5772, 1.9757) ccw
  line L95 (-48.6, -3.1) -> (-47.7792, -3.6518)
  line L96 (-54.9535, 8.1863) -> (-54.9535, 9.136)
  line L97 (-54.9535, 8.1863) -> (-53.2728, 7.2162)
  line L98 (-53.2728, 7.2162) -> (-53.2728, 5.1549)
  line L99 (-48.6, -3.1) -> (-48.5, 4.5)
  line L100 (-48.5, 4.5) -> (-50.6052, 5.6096)
  line L101 (-50.6052, 5.6096) -> (-50.6245, 4.1386)
  arc A14 (-53.2728, 5.1549) -> (-54.3, 3) centre (-52.5912, 3.5077) ccw
  arc A15 (-54.3, 3) -> (-52.3, 0) centre (-50.3, 3.5) ccw
  arc A16 (-52.3, 0) -> (-50.4, -0.2) centre (-51.1389, 1.9056) ccw
  arc A17 (-50.4, -0.2) -> (-49.6, 1.4) centre (-51.1365, 1.1682) ccw
  arc A18 (-49.6, 1.4) -> (-50.6245, 4.1386) centre (-53.5273, 1.4918) ccw
  constraint coincident A6 L78.end
  constraint coincident A6 L84.end
  constraint parallel L82 L84
  constraint coincident A6 L85.start
  constraint vertical L86
  constraint parallel L85 L87
  constraint horizontal L88
  constraint vertical L89
  constraint horizontal L90
  constraint vertical L91
  constraint coincident A6 L88.start
  constraint parallel L91 L93
  constraint parallel L92 L94
  constraint tangent A7 A9
  constraint tangent A11 A13
  constraint coincident A6 L95.end
  constraint parallel L78 L95
  constraint coincident A6 L96.end
  constraint perpendicular L90 L96
  constraint parallel L96 L98
  constraint parallel L99 L101
  constraint tangent A15 A17
extrude "Extrude3" cut sketch "Sketch3" against normal up to surface (3 mm away) contours A6 L95 L96 L97 L98 L99 L100 L101 A14 A15 A16 A17 A18 | A6 L78 L79 L80 L81 L82 L83 L84 E0 | A6 L85 L86 L87 L91 L92 L93 L94 A7 A8 A9 A10 A11 A12 A13
